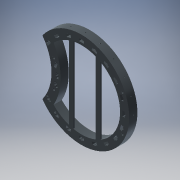
# Autodesk Inventor part: TSOP Plate
Saved by Autodesk Inventor 2016 (Build 200138000, 138)
## iProperties
Created: 2015-08-20
Part Number: TSOP Plate
Material: Iron, Gray
Document SubType Name: Modeling
Designer: TFHulbert
Density: 7.15 g/cm^3
Appearance: Iron Gray
Author: TFHulbert
Autodesk Inventor part; units mm, degrees
note: some values were not read from the file. Chosen so that the rebuilt part matches the saved one: direction of "Hole1"; copy form of "Circular Pattern1".
ref_plane "XZ Plane" through (0, 0, 0) normal (0, 1, 0) x (-1, 0, 0)
sketch "Sketch1" plane through (0, 0, 0) normal (0, 1, 0) x (-1, 0, 0)
  arc A0 (84.9551, 59.3682) -> (84.9503, 61.7126) centre (83.3322, 60.5371) ccw
  arc A1 (84.9551, 59.3682) -> (84.9551, -59.3682) centre (167.3819, 0) ccw
  arc A2 (84.9503, -61.7126) -> (84.9551, -59.3682) centre (83.3322, -60.5371) ccw
  circle A3 centre (60.8006, -30) radius 2.5
  circle A4 centre (60.8006, 30) radius 2.5
  arc A5 (84.9503, 61.7126) -> (84.9503, -61.7126) centre (0, 0) ccw
  arc A6 (61.1168, 59.074) -> (61.1168, -59.074) centre (167.3819, 0) ccw
  arc A7 (61.1168, 59.074) -> (61.1168, -59.074) centre (0, 0) ccw
  line L0 (-95.1231, 5.5) -> (-90.1231, 5.5)
  line L1 (-90.1231, 5.5) -> (-90.1231, -5.5)
  line L2 (-90.1231, -5.5) -> (-95.1231, -5.5)
  arc A8 (-95.1231, 2.5274) -> (-95.1231, -2.5274) centre (-94.1731, 0) ccw
  line L3 (-95.1231, -5.5) -> (-95.1231, -2.5274)
  line L4 (-95.1231, 2.5274) -> (-95.1231, 5.5)
  line L5 (-92.1671, -24.1638) -> (-87.4118, -22.6188)
  line L6 (-87.4118, -22.6188) -> (-84.0126, -33.0804)
  line L7 (-84.0126, -33.0804) -> (-88.7679, -34.6255)
  arc A9 (-91.2485, -26.991) -> (-89.6865, -31.7983) centre (-89.564, -29.1011) ccw
  line L8 (-88.7679, -34.6255) -> (-89.6865, -31.7983)
  line L9 (-91.2485, -26.991) -> (-92.1671, -24.1638)
  line L10 (-80.189, -51.4624) -> (-76.1439, -48.5234)
  line L11 (-76.1439, -48.5234) -> (-69.6783, -57.4226)
  line L12 (-69.6783, -57.4226) -> (-73.7234, -60.3616)
  arc A10 (-78.4418, -53.8673) -> (-75.4707, -57.9566) centre (-76.1876, -55.3536) ccw
  line L13 (-73.7234, -60.3616) -> (-75.4707, -57.9566)
  line L14 (-78.4418, -53.8673) -> (-80.189, -51.4624)
  line L15 (-60.3616, -73.7234) -> (-57.4226, -69.6783)
  line L16 (-57.4226, -69.6783) -> (-48.5234, -76.1439)
  line L17 (-48.5234, -76.1439) -> (-51.4624, -80.189)
  arc A11 (-57.9566, -75.4707) -> (-53.8673, -78.4418) centre (-55.3536, -76.1876) ccw
  line L18 (-51.4624, -80.189) -> (-53.8673, -78.4418)
  line L19 (-57.9566, -75.4707) -> (-60.3616, -73.7234)
  line L20 (-34.6255, -88.7679) -> (-33.0804, -84.0126)
  line L21 (-33.0804, -84.0126) -> (-22.6188, -87.4118)
  line L22 (-22.6188, -87.4118) -> (-24.1638, -92.1671)
  arc A12 (-31.7983, -89.6865) -> (-26.991, -91.2485) centre (-29.1011, -89.564) ccw
  line L23 (-24.1638, -92.1671) -> (-26.991, -91.2485)
  line L24 (-31.7983, -89.6865) -> (-34.6255, -88.7679)
  line L25 (-5.5, -95.1231) -> (-5.5, -90.1231)
  line L26 (-5.5, -90.1231) -> (5.5, -90.1231)
  line L27 (5.5, -90.1231) -> (5.5, -95.1231)
  arc A13 (-2.5274, -95.1231) -> (2.5274, -95.1231) centre (0, -94.1731) ccw
  line L28 (5.5, -95.1231) -> (2.5274, -95.1231)
  line L29 (-2.5274, -95.1231) -> (-5.5, -95.1231)
  line L30 (24.1638, -92.1671) -> (22.6188, -87.4118)
  line L31 (22.6188, -87.4118) -> (33.0804, -84.0126)
  line L32 (33.0804, -84.0126) -> (34.6255, -88.7679)
  arc A14 (26.991, -91.2485) -> (31.7983, -89.6865) centre (29.1011, -89.564) ccw
  line L33 (34.6255, -88.7679) -> (31.7983, -89.6865)
  line L34 (26.991, -91.2485) -> (24.1638, -92.1671)
  line L35 (51.4624, -80.189) -> (48.5234, -76.1439)
  line L36 (48.5234, -76.1439) -> (57.4226, -69.6783)
  line L37 (57.4226, -69.6783) -> (60.3616, -73.7234)
  arc A15 (53.8673, -78.4418) -> (57.9566, -75.4707) centre (55.3536, -76.1876) ccw
  line L38 (60.3616, -73.7234) -> (57.9566, -75.4707)
  line L39 (53.8673, -78.4418) -> (51.4624, -80.189)
  line L40 (71.2963, -58.5982) -> (67.2513, -55.6593)
  line L41 (67.2513, -55.6593) -> (73.7169, -46.7601)
  line L42 (73.7169, -46.7601) -> (77.762, -49.699)
  arc A16 (73.0436, -56.1933) -> (76.0147, -52.1039) centre (73.7606, -53.5902) ccw
  line L43 (77.762, -49.699) -> (76.0147, -52.1039)
  line L44 (73.0436, -56.1933) -> (71.2963, -58.5982)
  line L45 (57.1576, -24.3547) -> (52.4023, -22.8096)
  line L46 (52.4023, -22.8096) -> (55.8015, -12.348)
  line L47 (55.8015, -12.348) -> (60.5568, -13.893)
  arc A17 (58.0762, -21.5275) -> (59.6382, -16.7202) centre (57.9537, -18.8303) ccw
  line L48 (60.5568, -13.893) -> (59.6382, -16.7202)
  line L49 (58.0762, -21.5275) -> (57.1576, -24.3547)
  line L50 (55.5867, -5.5) -> (50.5867, -5.5)
  line L51 (50.5867, -5.5) -> (50.5867, 5.5)
  line L52 (50.5867, 5.5) -> (55.5867, 5.5)
  arc A18 (55.5867, -2.5274) -> (55.5867, 2.5274) centre (54.6367, 0) ccw
  line L53 (55.5867, 5.5) -> (55.5867, 2.5274)
  line L54 (55.5867, -2.5274) -> (55.5867, -5.5)
  line L55 (60.5568, 13.893) -> (55.8015, 12.348)
  line L56 (55.8015, 12.348) -> (52.4023, 22.8096)
  line L57 (52.4023, 22.8096) -> (57.1576, 24.3547)
  arc A19 (59.6382, 16.7202) -> (58.0762, 21.5275) centre (57.9537, 18.8303) ccw
  line L58 (57.1576, 24.3547) -> (58.0762, 21.5275)
  line L59 (59.6382, 16.7202) -> (60.5568, 13.893)
  line L60 (77.762, 49.699) -> (73.7169, 46.7601)
  line L61 (73.7169, 46.7601) -> (67.2513, 55.6593)
  line L62 (67.2513, 55.6593) -> (71.2963, 58.5982)
  arc A20 (76.0147, 52.1039) -> (73.0436, 56.1933) centre (73.7606, 53.5902) ccw
  line L63 (71.2963, 58.5982) -> (73.0436, 56.1933)
  line L64 (76.0147, 52.1039) -> (77.762, 49.699)
  line L65 (60.3616, 73.7234) -> (57.4226, 69.6783)
  line L66 (57.4226, 69.6783) -> (48.5234, 76.1439)
  line L67 (48.5234, 76.1439) -> (51.4624, 80.189)
  arc A21 (57.9566, 75.4707) -> (53.8673, 78.4418) centre (55.3536, 76.1876) ccw
  line L68 (51.4624, 80.189) -> (53.8673, 78.4418)
  line L69 (57.9566, 75.4707) -> (60.3616, 73.7234)
  line L70 (34.6255, 88.7679) -> (33.0804, 84.0126)
  line L71 (33.0804, 84.0126) -> (22.6188, 87.4118)
  line L72 (22.6188, 87.4118) -> (24.1638, 92.1671)
  arc A22 (31.7983, 89.6865) -> (26.991, 91.2485) centre (29.1011, 89.564) ccw
  line L73 (24.1638, 92.1671) -> (26.991, 91.2485)
  line L74 (31.7983, 89.6865) -> (34.6255, 88.7679)
  line L75 (5.5, 95.1231) -> (5.5, 90.1231)
  line L76 (5.5, 90.1231) -> (-5.5, 90.1231)
  line L77 (-5.5, 90.1231) -> (-5.5, 95.1231)
  arc A23 (2.5274, 95.1231) -> (-2.5274, 95.1231) centre (0, 94.1731) ccw
  line L78 (-5.5, 95.1231) -> (-2.5274, 95.1231)
  line L79 (2.5274, 95.1231) -> (5.5, 95.1231)
  line L80 (-24.1638, 92.1671) -> (-22.6188, 87.4118)
  line L81 (-22.6188, 87.4118) -> (-33.0804, 84.0126)
  line L82 (-33.0804, 84.0126) -> (-34.6255, 88.7679)
  arc A24 (-26.991, 91.2485) -> (-31.7983, 89.6865) centre (-29.1011, 89.564) ccw
  line L83 (-34.6255, 88.7679) -> (-31.7983, 89.6865)
  line L84 (-26.991, 91.2485) -> (-24.1638, 92.1671)
  line L85 (-51.4624, 80.189) -> (-48.5234, 76.1439)
  line L86 (-48.5234, 76.1439) -> (-57.4226, 69.6783)
  line L87 (-57.4226, 69.6783) -> (-60.3616, 73.7234)
  arc A25 (-53.8673, 78.4418) -> (-57.9566, 75.4707) centre (-55.3536, 76.1876) ccw
  line L88 (-60.3616, 73.7234) -> (-57.9566, 75.4707)
  line L89 (-53.8673, 78.4418) -> (-51.4624, 80.189)
  line L90 (-73.7234, 60.3616) -> (-69.6783, 57.4226)
  line L91 (-69.6783, 57.4226) -> (-76.1439, 48.5234)
  line L92 (-76.1439, 48.5234) -> (-80.189, 51.4624)
  arc A26 (-75.4707, 57.9566) -> (-78.4418, 53.8673) centre (-76.1876, 55.3536) ccw
  line L93 (-80.189, 51.4624) -> (-78.4418, 53.8673)
  line L94 (-75.4707, 57.9566) -> (-73.7234, 60.3616)
  line L95 (-88.7679, 34.6255) -> (-84.0126, 33.0804)
  line L96 (-84.0126, 33.0804) -> (-87.4118, 22.6188)
  line L97 (-87.4118, 22.6188) -> (-92.1671, 24.1638)
  arc A27 (-89.6865, 31.7983) -> (-91.2485, 26.991) centre (-89.564, 29.1011) ccw
  line L98 (-92.1671, 24.1638) -> (-91.2485, 26.991)
  line L99 (-89.6865, 31.7983) -> (-88.7679, 34.6255)
  line L100 (76.1876, -55.3536) -> (73.7606, -53.5902)
  arc A28 (84.9551, 59.3682) -> (84.9503, 61.7126) centre (83.3322, 60.5371) ccw
  arc A29 (84.9551, 59.3682) -> (84.9551, -59.3682) centre (167.3819, 0) ccw
  arc A30 (84.9503, -61.7126) -> (84.9551, -59.3682) centre (83.3322, -60.5371) ccw
  arc A31 (21.6511, 102.7435) -> (-99.804, 32.6214) centre (0, 0) ccw
  arc A32 (-99.804, -32.6214) -> (21.6511, -102.7435) centre (0, 0) ccw
  circle A33 centre (-90, -40) radius 2.5
  line L101 (-90.1231, 0) -> (-96.8731, 0)
  circle A34 centre (-90, 40) radius 2.5
  point P0 (-105, 0)
  dimension "d11" = 360
  dimension "d15" = 3
  dimension "d90" = 5
  dimension "d104" = 90
  dimension "d105" = 40
  dimension "d106" = 90
  dimension "d107" = 40
  constraints: 204 end point, 64 point on circle, 35 centre point, 3 perpendicular, 1 horizontal, 1 midpoint, 1 symmetric about line, 185 other
  measures "d15" distance of L100.start L100.end
  measures "d90" diameter of A33
  measures "d104" horizontal distance of A34.centre point (0, 0)
  measures "d105" vertical distance of point (0, 0) A34.centre
  measures "d106" horizontal distance of A32.centre A33.centre
  measures "d107" vertical distance of point (0, 0) A33.centre
extrude "Extrusion1" add sketch "Sketch1" along normal blind 18 contours A1 A2 A5 A0 | A3 | A4 | L0 L1 L101 A8 L4 | L1 L2 L3 A8 L101 | L5 L6 L7 L8 A9 L9 | L10 L11 L12 L13 A10 L14 | L15 L16 L17 L18 A11 L19 | L20 L21 L22 L23 A12 L24 | L25 L26 L27 L28 A13 L29 | L30 L31 L32 L33 A14 L34 | L35 L36 L37 L38 A15 L39 | L40 L41 L42 L43 A16 L44 | L45 L46 L47 L48 A17 L49 | L50 L51 L52 L53 A18 L54 | L55 L56 L57 L58 A19 L59 | L60 L61 L62 L63 A20 L64 | L65 L66 L67 L68 A21 L69 | L70 L71 L72 L73 A22 L74 | L75 L76 L77 L78 A23 L79 | L80 L81 L82 L83 A24 L84 | L85 L86 L87 L88 A25 L89 | L90 L91 L92 L93 A26 L94 | L95 L96 L97 L98 A27 L99 | A33 | A34
extrude "Extrusion2" cut sketch "Sketch1" along normal through all contours A3 | A4
extrude "Extrusion3" cut sketch "Sketch1" along normal blind 12.6 contours L0 L1 L101 A8 L4 | L1 L2 L3 A8 L101 | L5 L6 L7 L8 A9 L9 | L10 L11 L12 L13 A10 L14 | L15 L16 L17 L18 A11 L19 | L20 L21 L22 L23 A12 L24 | L25 L26 L27 L28 A13 L29 | L30 L31 L32 L33 A14 L34 | L35 L36 L37 L38 A15 L39 | L40 L41 L42 L43 A16 L44 | L45 L46 L47 L48 A17 L49 | L50 L51 L52 L53 A18 L54 | L55 L56 L57 L58 A19 L59 | L60 L61 L62 L63 A20 L64 | L65 L66 L67 L68 A21 L69 | L70 L71 L72 L73 A22 L74 | L75 L76 L77 L78 A23 L79 | L80 L81 L82 L83 A24 L84 | L85 L86 L87 L88 A25 L89 | L90 L91 L92 L93 A26 L94 | L95 L96 L97 L98 A27 L99
ref_plane "Work Plane3" through (105, 0, 0) normal (1, 0, 0) x (0, 1, 0)
sketch "Sketch2" plane through (105, 0, 0) normal (1, 0, 0) x (0, 1, 0)
  line L0 (0, 0) -> (9.2, 0)
  circle A0 centre (9.2, 0) radius 2
  dimension "d29" = 9.2
  dimension "d30" = 4
  constraints: 2 end point, 1 centre point, 1 coincident, 1 horizontal
  measures "d29" distance of L0.start L0.end
  measures "d30" diameter of A0
hole "Hole1" at (105, 9.2, 0) direction (-1, 0, 0) diameter 2 end up to surface
pattern_circular "Circular Pattern1" count 20 over 360 about axis through (0, -10, 0) along (0, 1, 0) of "Hole1" geometry pattern yes
ref_plane "Work Plane4" through (-54.1019, 0, 17.5788) normal (-0.9510565, 0, 0.309017) x (0.309017, 0, 0.9510565)
sketch "Sketch3" plane through (-54.1019, 0, 17.5788) normal (-0.9510565, 0, 0.309017) x (0.309017, 0, 0.9510565)
  line L0 (0, 0) -> (0, 9.2)
  circle A0 centre (0, 9.2) radius 2
  dimension "d41" = 9.2
  dimension "d42" = 4
  constraints: 2 end point, 1 centre point, 1 coincident, 1 vertical
  measures "d41" distance of L0.start L0.end
  measures "d42" diameter of A0
hole "Hole2" at (-54.1019, 9.2, 17.5788) direction (-0.9510565, 0, 0.309017) diameter 2 end up to surface
sketch "Sketch4" plane through (-50.5867, 0, 5.5) normal (-1, 0, 0) x (0, 0, 1)
  line L0 (-5.5, 0) -> (-5.5, 9.2)
  circle A0 centre (-5.5, 9.2) radius 2
  dimension "d51" = 9.2
  dimension "d52" = 4
  constraints: 2 end point, 1 centre point, 1 coincident, 1 vertical
  measures "d51" distance of L0.start L0.end
  measures "d52" diameter of A0
hole "Hole3" at (-50.5867, 9.2, 0) direction (-1, 0, 0) diameter 2 end up to surface
mirror "Mirror1" about plane through (0, 0, 0) normal (0, 0, 1) of "Hole2"
extrude "Extrusion10" cut sketch "Sketch1" along normal through all contours A33 | A34
sketch "Sketch13" plane through (0, 0, 0) normal (0, -1, 0) x (1, 0, 0)
  arc A0 (-17.7978, 83.1158) -> (-27.436, 80.4504) centre (0, 0) ccw projected
  line L0 (-27.436, -80.4504) -> (-27.436, 80.4504) projected
  line L1 (-27.436, 80.4504) -> (-27.436, -80.4504)
  line L2 (-17.7978, -83.1158) -> (-17.7978, 83.1158) projected
  line L3 (-17.7978, -83.1158) -> (-17.7978, 83.1158)
  line L4 (31.4817, -78.9551) -> (31.4817, 78.9551) projected
  line L5 (31.4817, 78.9551) -> (31.4817, -78.9551)
  line L6 (41.4817, 74.1908) -> (41.4817, -74.1908) projected
  line L7 (41.4817, 74.1908) -> (41.4817, -74.1908)
  line L8 (-27.436, -80.4504) -> (-27.436, -83.1158)
  line L9 (-27.436, -83.1158) -> (-17.7978, -83.1158)
  line L10 (31.4817, -78.9551) -> (31.4817, -80.4504)
  line L11 (31.4817, -80.4504) -> (41.4817, -75.3798)
  line L12 (41.4817, -75.3798) -> (41.4817, -74.1908)
  arc A1 (-61.1168, -59.074) -> (-61.1168, 59.074) centre (0, 0) ccw projected
  line L13 (31.4817, 78.9551) -> (31.4817, 81.2461)
  line L14 (31.4817, 81.2461) -> (41.4817, 74.1908)
  line L15 (-27.436, 80.4504) -> (-27.436, 83.7291)
  line L16 (-27.436, 83.7291) -> (-17.7978, 83.1158)
  constraints: 26 end point, 5 vertical, 2 collinear, 1 perpendicular, 1 point on line, 2 other
extrude "Extrusion11" add sketch "Sketch13" against normal blind 3 contours L2 A1 L0 A0 | A1 L6 L4
ref_plane "Work Plane6" through (0, 0, 0) normal (0, 0, 1) x (1, 0, 0)
body "Solid1"
